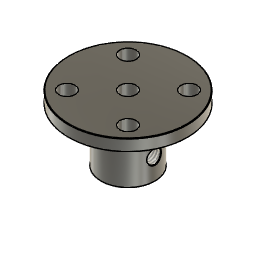
Motor_Holder v1 (Autodesk Fusion 360 design; units mm, degrees)
Autodesk Fusion 360 part; units mm, degrees
note: some values were not read from the file. Set by a fixed rule: the direction of a hole.
sketch "Sketch1" plane through (0, 0, 0) normal (0, 0, 1) x (1, 0, 0)
  line L0 (-5.65, 5.65) -> (5.65, 5.65) construction
  line L1 (5.65, 5.65) -> (5.65, -5.65) construction
  line L2 (5.65, -5.65) -> (-5.65, -5.65) construction
  line L3 (-5.65, -5.65) -> (-5.65, 5.65) construction
  line L4 (-5.65, 5.65) -> (5.65, -5.65) construction
  line L5 (5.65, 5.65) -> (-5.65, -5.65) construction
  circle A0 centre (0, 0) radius 11
  point P0 (-5.65, 5.65)
  point P1 (5.65, 5.65)
  point P2 (5.65, -5.65)
  point P3 (-5.65, -5.65)
  dimension "d1" = 11.3
  dimension "d2" = 22
  constraint horizontal L0
  constraint perpendicular L0 L1
  constraint parallel L0 L2
  constraint parallel L1 L3
  constraint coincident L4 A0.centre
  constraint coincident L5 A0.centre
  constraint coincident A0.centre origin
  constraint equal L0 L3
  constraint coincident P0 L0.start
  constraint coincident P1 L0.end
  constraint coincident P2 L1.end
  constraint coincident P3 L2.end
  measures "d1" distance of P0 P3
  measures "d2" diameter of A0
extrude "Extrude1" add sketch "Sketch1" along normal blind 2.2
sketch "Sketch2" plane through (0, 0, 0) normal (0, 0, -1) x (1, 0, 0)
  circle A0 centre (0, 0) radius 5
  dimension "d5" = 10
  constraint coincident A0.centre origin
  measures "d5" diameter of A0
extrude "Extrude2" add sketch "Sketch2" along normal blind 10
hole "Hole1" at (0, 0, 2.2) direction (0, 0, -1) diameter 3 depth 12.7 tip angle 118
hole "Hole2" at (5.65, 5.65, 0) at (-5.65, 5.65, 0) at (-5.65, -5.65, 0) at (5.65, -5.65, 0) direction (0, 0, 1) diameter 3 depth 12.7 tip angle 118
chamfer "Chamfer1" distance 0.1 angle 45 1 edges at (-4.6616, 1.8081, -10)
chamfer "Chamfer1" distance 0.1 angle 45 2 edges at (-10.2556, -3.9778, 0) (-10.2556, -3.9778, 2.2)
chamfer "Chamfer1" distance 0.1 angle 45 1 edges at (-4.6616, -1.8081, 0)
sketch "Sketch3" plane through (0, 0, 0) normal (1, 0, 0) x (0, 1, 0)
  line L0 (0, -10) -> (0, -6) construction
  point P0 (0, -10)
  dimension "d17" = 4
  constraint coincident P0 L0.start
  constraint vertical L0
  measures "d17" distance of P0 L0.end
ref_plane "WorkPlane1" through (-5, 0, -5) normal (-1, 0, 0) x (0, 1, 0)
sketch "Sketch4" plane through (-5, 0, 0) normal (-1, 0, 0) x (0, -1, 0)
  point P0 (0, -6)
hole "Hole3" at (-5, 0, -6) direction (1, 0, 0) diameter 2.54 depth 12.7 tip angle 118
thread "Thread1" "ANSI Metric M Profile 3.0 M3x0.5 6H" thread offset 0 thread depth 5.9436
chamfer "Chamfer2" distance 0.1 angle 45 4 edges at (-5, 0.009, -7.27) (4.836, 1.27, -6.009) (-5, 0.009, -7.27) (4.836, 1.27, -6.009)
